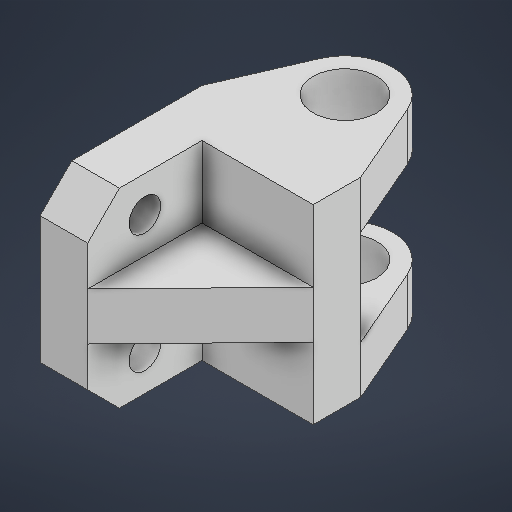
# Autodesk Inventor part: 01
Saved by Autodesk Inventor 2025.1 (Build 291241020, 241B)
## iProperties
Created: 2026-04-19
Part Number: 01
Material: Generic
Document SubType Name: Modeling
Designer: Tolin
Density: 1 g/cm^3
Appearance: Default
Author: Tolin
Autodesk Inventor part; units mm, degrees
ref_plane "YZ Plane" through (0, 0, 0) normal (1, 0, 0) x (0, 1, 0)
sketch "Sketch1" plane through (0, 0, 0) normal (0, 0, 1) x (1, 0, 0)
  line L0 (0, 60) -> (50, 60)
  line L1 (50, 60) -> (50, 0)
  line L2 (50, 0) -> (0, 0)
  line L3 (0, 0) -> (0, 60)
  dimension "d0" = 50
  dimension "d1" = 60
  constraints: 8 end point, 2 parallel, 1 coincident, 1 horizontal, 1 perpendicular
  measures "d0" distance between parallel lines of L1 L3
  measures "d1" distance between parallel lines of L0 L2
extrude "Extrusion1" add sketch "Sketch1" along normal blind 15
sketch "Sketch2" plane through (0, 60, 0) normal (0, 1, 0) x (1, 0, 0)
  circle A0 centre (25, 20) radius 10
  circle A1 centre (25, 20) radius 15
  line L0 (50, 0) -> (0, 0) projected
  line L1 (25, 0) -> (25, 35.9147) construction
  line L2 (0, 0) -> (0, -15) construction
  line L3 (0, 0) -> (11.2339, 25.9577)
  line L4 (50, 0) -> (50, -15) projected
  line L5 (50, 0) -> (38.7661, 25.9577)
  dimension "d4" = 20
  dimension "d5" = 30
  dimension "d6" = 20
  constraints: 6 end point, 2 centre point, 2 point on circle, 2 tangent, 1 coincident, 1 midpoint, 1 point on line, 1 vertical
  measures "d4" diameter of A0
  measures "d5" diameter of A1
  measures "d6" distance from line of L0 A0.centre
extrude "Extrusion2" add sketch "Sketch2" against normal blind 15
ref_plane "Work Plane1" through (0, 30, 15) normal (0, 1, 0) x (1, 0, 0)
mirror "Mirror1" about plane through (0, 30, 15) normal (0, 1, 0) of "Extrusion2"
sketch "Sketch3" plane through (0, 0, 15) normal (0, 0, 1) x (1, 0, 0)
  line L0 (50, 0) -> (50, 60) projected
  line L1 (0, 60) -> (0, 0) projected
  line L2 (50, 60) -> (0, 60) projected
  line L3 (0, 0) -> (15, 0)
  line L4 (15, 0) -> (15, 60)
  line L5 (15, 60) -> (0, 60)
  line L6 (0, 60) -> (0, 0)
  dimension "d12" = 15
  constraints: 8 end point, 2 parallel, 1 horizontal, 1 perpendicular, 1 point on line
  measures "d12" distance between parallel lines of L1 L4
extrude "Extrusion3" add sketch "Sketch3" along normal blind 36
ref_plane "Work Plane3" through (15, 22.5, 51) normal (0, -1, 0) x (0, 0, -1)
sketch "Sketch5" plane through (15, 22.5, 51) normal (0, -1, 0) x (0, 0, -1)
  line L0 (36, 0) -> (0, 0) projected
  line L1 (0, 0) -> (36, 35)
  line L2 (36, 0) -> (36, 35)
  point P0 (51, -15)
  constraints: 4 end point, 1 vertical
extrude "Extrusion4" add sketch "Sketch5" against normal blind 15
chamfer "Chamfer1" distance 10 angle 45 2 edges at (7.5, 0, 51) (7.5, 60, 51)
sketch "Sketch7" plane through (15, 37.5, 15) normal (1, 0, 0) x (0, 0, -1)
  line L0 (0, 22.5) -> (-26, 22.5) projected
  line L1 (-36, 0) -> (0, 0) projected
  line L2 (0, 0) -> (0, 22.5) projected
  line L3 (-36, 0) -> (-36, 12.5) projected
  line L4 (-5.5947, -7.5) -> (-36, -7.5) construction
  line L5 (-36, 12.5) -> (-36, -27.5) construction
  point P0 (15, -37.5)
  point P1 (-18, 11.25)
  point P2 (-18, -26.25)
  dimension "d28" = 11.25
  dimension "d29" = 22.5
  dimension "d30" = 36
  dimension "d31" = 18
  constraints: 2 end point, 1 horizontal, 1 midpoint, 1 symmetric about line
  measures "d28" distance from line of L0 point (-18, 11.25)
  measures "d29" distance between parallel lines of L0 L1
  measures "d30" distance between parallel lines of L2 L3
  measures "d31" distance from line of L2 point (-18, 11.25)
hole "Hole2" at (15, 48.75, 33) at (15, 11.25, 33) direction (-1, 0, 0) diameter 10 end through all
equation "\"d28\" = 0.5 * d29"
equation "\"d31\" = 0.5 * d30"
body "Solid1"
